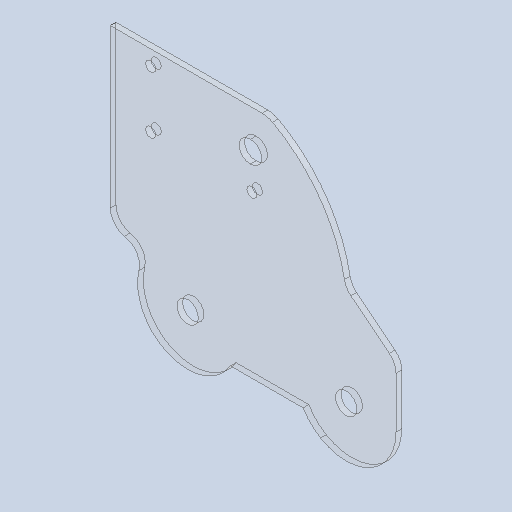
# Autodesk Inventor part: Intake Sides V4_bearing
Saved by Autodesk Inventor 2022 (Build 260153000, 153)
## iProperties
Created: 2022-10-16
Part Number: Intake Sides V4_bearing
Material: Polycarbonate, Clear
Document SubType Name: Modeling
Designer: matt
Density: 1.2 g/cm^3
Appearance: Polycarbonate - Clear
Mass: 66.752 g
Surface Area: 373.255 cm^2
Volume: 55.6267 cm^3
Author: matt
Autodesk Inventor part; units mm, degrees
ref_plane "YZ Plane" through (0, 0, 0) normal (1, 0, 0) x (0, 1, 0)
ref_plane "XZ Plane" through (0, 0, 0) normal (0, 1, 0) x (-1, 0, 0)
ref_plane "XY Plane" through (0, 0, 0) normal (0, 0, 1) x (1, 0, 0)
sketch "Sketch1" plane through (0, 0, 0) normal (0, 0, 1) x (1, 0, 0)
  line L0 (90.4273, 0.002) -> (0, 0.002)
  line L1 (0, 0.002) -> (0, -88.6441)
  arc A0 (0, -88.6441) -> (7.9382, -98.4293) centre (10, -88.6441) ccw
  arc A1 (16.0457, -111.012) -> (7.9382, -98.4293) centre (6.4076, -108.3189) ccw
  arc A2 (145.7944, -114.2869) -> (148.0953, -110.4201) centre (146.9707, -112.3688) ccw
  circle A3 centre (97.4707, -122.3689) radius 2.25
  circle A4 centre (97.4707, -112.3689) radius 2.25
  circle A5 centre (78.1758, -122.3689) radius 2.25
  arc A6 (145.7944, -124.2869) -> (148.0953, -120.4201) centre (146.9707, -122.3689) ccw
  circle A7 centre (22.6171, -8.5119) radius 2.8
  circle A8 centre (22.6171, -40.5119) radius 2.8
  circle A9 centre (28.6758, -122.3689) radius 2.25
  circle A10 centre (28.6758, -112.3689) radius 2.25
  circle A11 centre (78.1758, -112.3689) radius 2.25
  circle A12 centre (78.9344, -21.998) radius 3.25
  circle A13 centre (10, -90.6616) radius 3.3
  line L2 (73.0605, -128.2915) -> (33.527, -128.2915)
  arc A14 (32.527, -127.2915) -> (33.527, -128.2915) centre (33.527, -127.2915) ccw
  line L3 (32.527, -127.2915) -> (32.527, -107.4915)
  arc A15 (33.527, -106.4915) -> (32.527, -107.4915) centre (33.527, -107.4915) ccw
  line L4 (33.527, -106.4915) -> (73.0605, -106.4915)
  arc A16 (74.0605, -107.4915) -> (73.0605, -106.4915) centre (73.0605, -107.4915) ccw
  line L5 (74.0605, -107.4915) -> (74.0605, -127.2915)
  arc A17 (73.0605, -128.2915) -> (74.0605, -127.2915) centre (73.0605, -127.2915) ccw
  line L6 (142.1195, -128.2915) -> (102.586, -128.2915)
  arc A18 (101.586, -127.2915) -> (102.586, -128.2915) centre (102.586, -127.2915) ccw
  line L7 (101.586, -127.2915) -> (101.586, -107.4915)
  arc A19 (102.586, -106.4915) -> (101.586, -107.4915) centre (102.586, -107.4915) ccw
  line L8 (102.586, -106.4915) -> (142.1195, -106.4915)
  arc A20 (143.1195, -107.4915) -> (142.1195, -106.4915) centre (142.1195, -107.4915) ccw
  line L9 (143.1195, -107.4915) -> (143.1195, -127.2915)
  arc A21 (142.1195, -128.2915) -> (143.1195, -127.2915) centre (142.1195, -127.2915) ccw
  circle A22 centre (146.9707, -112.3688) radius 2.25
  circle A23 centre (146.9707, -122.3689) radius 2.25
  line L10 (28.6758, -112.3689) -> (146.9707, -112.3688) construction
  line L11 (28.6758, -122.3689) -> (146.9707, -122.3689) construction
  circle A24 centre (43.3732, -117.3689) radius 5.9 construction
  circle A25 centre (132.2732, -117.3688) radius 5.9 construction
  circle A26 centre (43.3732, -117.3689) radius 6
  circle A27 centre (132.2732, -117.3688) radius 6
  line L12 (10, -90.6616) -> (176.2125, -90.6616) construction
  circle A28 centre (78.9344, -21.998) radius 6
  circle A29 centre (79.375, -41.275) radius 2.8
  line L13 (0.0516, 0) -> (0, 0) projected
  line L14 (0, 0) -> (0, -88.6441) projected
  arc A30 (0, -88.6441) -> (8.2038, -98.4815) centre (10, -88.6441) ccw projected
  arc A31 (16.1218, -110.6924) -> (8.2038, -98.4815) centre (6.4076, -108.3189) ccw projected
  arc A32 (16.1218, -110.6924) -> (67.3839, -131.6564) centre (43.3217, -117.3382) ccw projected
  line L15 (67.3839, -131.6564) -> (108.1595, -131.6564) projected
  arc A33 (108.1595, -131.6564) -> (117.931, -141.4167) centre (132.2217, -117.3382) ccw projected
  arc A34 (117.931, -141.4167) -> (160.2733, -117.3688) centre (132.2732, -117.3688) ccw projected
  line L16 (160.2733, -117.3688) -> (160.2733, -88.8237) projected
  arc A35 (160.2733, -88.8237) -> (156.504, -81.0021) centre (150.2733, -88.8237) ccw projected
  line L17 (156.504, -81.0021) -> (134.9366, -63.8213) projected
  arc A36 (131.3222, -57.7523) -> (134.9366, -63.8213) centre (141.1674, -55.9997) ccw projected
  arc A37 (131.3222, -57.7523) -> (90.9953, -1.4859) centre (52.2705, -71.825) ccw projected
  arc A38 (90.9953, -1.4859) -> (85.2079, 0.002) centre (85.2079, -11.998) ccw projected
  line L18 (85.2079, 0.002) -> (0.0516, 0.002) projected
  line L19 (0.0516, 0.002) -> (0.0516, 0) projected
  circle A39 centre (155.0516, -88.6441) radius 3.3 projected
  line L20 (102.586, -106.4915) -> (142.1195, -106.4915) projected
  arc A40 (143.1195, -107.4915) -> (142.1195, -106.4915) centre (142.1195, -107.4915) ccw projected
  line L21 (143.1195, -107.4915) -> (143.1195, -127.2915) projected
  arc A41 (142.1195, -128.2915) -> (143.1195, -127.2915) centre (142.1195, -127.2915) ccw projected
  line L22 (142.1195, -128.2915) -> (102.586, -128.2915) projected
  arc A42 (101.586, -127.2915) -> (102.586, -128.2915) centre (102.586, -127.2915) ccw projected
  line L23 (101.586, -127.2915) -> (101.586, -107.4915) projected
  arc A43 (102.586, -106.4915) -> (101.586, -107.4915) centre (102.586, -107.4915) ccw projected
  line L24 (74.0605, -107.4915) -> (74.0605, -127.2915) projected
  arc A44 (73.0605, -128.2915) -> (74.0605, -127.2915) centre (73.0605, -127.2915) ccw projected
  line L25 (73.0605, -128.2915) -> (33.527, -128.2915) projected
  arc A45 (32.527, -127.2915) -> (33.527, -128.2915) centre (33.527, -127.2915) ccw projected
  line L26 (32.527, -127.2915) -> (32.527, -107.4915) projected
  arc A46 (33.527, -106.4915) -> (32.527, -107.4915) centre (33.527, -107.4915) ccw projected
  line L27 (33.527, -106.4915) -> (73.0605, -106.4915) projected
  arc A47 (74.0605, -107.4915) -> (73.0605, -106.4915) centre (73.0605, -107.4915) ccw projected
  circle A48 centre (28.6758, -112.3689) radius 2.25 projected
  circle A49 centre (28.6758, -122.3689) radius 2.25 projected
  circle A50 centre (78.1758, -21.998) radius 6 projected
  circle A51 centre (78.1758, -122.3689) radius 2.25 projected
  circle A52 centre (97.4707, -112.3689) radius 2.25 projected
  circle A53 centre (146.9707, -112.3688) radius 2.25 projected
  circle A54 centre (146.9707, -122.3689) radius 2.25 projected
  circle A55 centre (22.6171, -8.5119) radius 2.8 projected
  circle A56 centre (22.6171, -40.5119) radius 2.8 projected
  circle A57 centre (97.4707, -122.3689) radius 2.25 projected
  circle A58 centre (78.1758, -112.3689) radius 2.25 projected
  circle A59 centre (10, -88.6441) radius 3.3 projected
  point P0 (0, 0)
  point P1 (58.8546, -117.3689)
  point P2 (148.0953, -110.4201)
  point P3 (151.6186, -98.07)
  point P4 (85.2079, 0.002)
  point P5 (13.142, -89.6529)
  point P6 (6.858, -89.6529)
  point P7 (78.5551, -27.986)
  point P8 (78.5551, -16.01)
  dimension "d2" = 49.5
  dimension "d3" = 49.5
  dimension "d4" = 49.5
  dimension "d5" = 49.5
  dimension "d6" = 10
  dimension "d7" = 12
  dimension "d8" = 12
  dimension "d9" = 6.6
  dimension "d10" = 10
  dimension "d12" = 10
  dimension "d16" = 12
  dimension "d17" = 5.6
  dimension "d18" = 22
  constraints: 28 centre point, 26 end point, 25 point on circle, 5 coincident, 4 concentric, 4 point on line, 2 collinear, 2 horizontal, 1 perpendicular
  measures "d2" distance of A11.centre L10.start
  measures "d3" distance of A5.centre L11.start
  measures "d4" distance of L11.end A3.centre
  measures "d5" distance of L10.end A4.centre
  measures "d6" distance of L11.start L10.start
  measures "d7" diameter of A26
  measures "d8" diameter of A27
  measures "d9" diameter of A13
  measures "d10" distance from line of L1 L12.start
  measures "d12" radius of A0
  measures "d16" diameter of A28
  measures "d17" diameter of A29
  measures "d18" distance from line of A28.centre L0
extrude "Extrusion1" add sketch "Sketch1" along normal blind 3.175 contours A38 A37 A36 L17 A35 L16 A34 A33 L15 A32 A1 A0 L1 L0 | A22 A2 | A3 | A4 | A5 | A23 A6 | A9 | A10 | A11 | A13 A59 | A59 A13 | A13 A59 | L2 A14 L3 A15 L4 A16 L5 A17 | L6 A18 L7 A19 L8 A20 L9 A21 | A39
body "Solid1"
